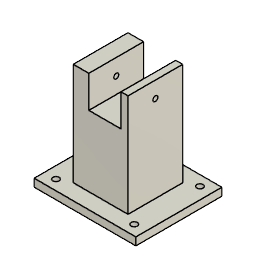
Base_Frotal (Autodesk Fusion 360 design; units mm, degrees)
Autodesk Fusion 360 part; units mm, degrees
sketch "Boceto2" plane through (0, 0, 0) normal (0, 0, 1) x (1, 0, 0)
  line L0 (0, 0) -> (35, 0)
  line L1 (35, 0) -> (35, 35)
  line L2 (35, 35) -> (0, 35)
  line L3 (0, 35) -> (0, 0)
  line L4 (50, -10) -> (-15, -10)
  line L5 (-15, -10) -> (-15, 45)
  line L6 (-15, 45) -> (50, 45)
  line L7 (50, 45) -> (50, -10)
  line L8 (50, -10) -> (-15, 45) construction
  line L9 (-15, -10) -> (50, 45) construction
  line L10 (42.5, 38.5) -> (-7.5, 38.5) construction
  line L11 (-7.5, 38.5) -> (-7.5, -3.5) construction
  line L12 (-7.5, -3.5) -> (42.5, -3.5) construction
  line L13 (42.5, -3.5) -> (42.5, 38.5) construction
  line L14 (42.5, 38.5) -> (-7.5, -3.5) construction
  line L15 (-7.5, 38.5) -> (42.5, -3.5) construction
  circle A0 centre (42.5, 38.5) radius 2
  line L16 (17.5, 45) -> (17.5, -10) construction
  line L17 (-15, 17.5) -> (50, 17.5) construction
  circle A1 centre (-7.5, 38.5) radius 2
  circle A2 centre (-7.5, -3.5) radius 2
  circle A3 centre (42.5, -3.5) radius 2
  point P0 (17.5, 17.5)
  point P1 (17.5, 17.5)
  dimension "d8" = 35
  dimension "d9" = 35
  dimension "d10" = 15
  dimension "d12" = 10
  dimension "d13" = 10
  dimension "d14" = 15
  dimension "d15" = 50
  dimension "d16" = 42
  dimension "d17" = 4
  constraint horizontal L0
  constraint vertical L1
  constraint horizontal L2
  constraint vertical L3
  constraint coincident L0.start L3.end
  constraint horizontal L4
  constraint perpendicular L4 L5
  constraint parallel L4 L6
  constraint parallel L5 L7
  constraint coincident L8 P1
  constraint coincident L9 P1
  constraint horizontal L10
  constraint perpendicular L10 L11
  constraint parallel L10 L12
  constraint parallel L11 L13
  constraint coincident L14 P1
  constraint coincident L15 P1
  constraint coincident P1 P0
  constraint coincident L10.start L13.end
  constraint midpoint L6 L16.start
  constraint midpoint L4 L16.end
  constraint midpoint L5 L17.start
  constraint midpoint L7 L17.end
  constraint symmetric A0 L16 A1
  constraint symmetric A0 L17 A3
  constraint symmetric L17 A1 A2
  measures "d8" distance of L0 L2
  measures "d9" distance of L1 L3
  measures "d10" distance of L3 L5
  measures "d12" distance of L0 L4
  measures "d13" distance of L2 L6
  measures "d14" distance of L1 L7
  measures "d15" distance of L11.end L12.end
  measures "d16" distance of L10.end L11.end
  measures "d17" diameter of A0
extrude "Extruir1" add sketch "Boceto2" along normal blind 70.5 contours L0 L1 L2 L3
sketch "Boceto3" plane through (0, 0, 0) normal (0, -1, 0) x (1, 0, 0)
  line L0 (0, 0) -> (35, 0)
  line L1 (35, 0) -> (35, 70.5)
  line L2 (35, 70.5) -> (0, 70.5)
  line L3 (0, 70.5) -> (0, 0)
  line L4 (0, 70.5) -> (10, 70.5)
  line L5 (10, 70.5) -> (30.5, 70.5)
  line L6 (30.5, 70.5) -> (30.5, 50)
  line L7 (30.5, 50) -> (10, 50)
  line L8 (10, 50) -> (10, 70.5)
  dimension "d3" = 10
  dimension "d4" = 20.5
  dimension "d5" = 20.5
  constraint coincident L2.end L3.start
  constraint perpendicular L1 L4
  constraint horizontal L5
  constraint vertical L6
  constraint horizontal L7
  constraint vertical L8
  measures "d3" distance of L2.end L4.end
  measures "d4" distance of L4.end L5.end
  measures "d5" distance of L4.end L7.end
extrude "Extruir2" cut sketch "Boceto3" against normal blind 35 contours L2 L5 L6 L7 L8
sketch "Boceto4" plane through (0, 0, 50) normal (0, 0, 1) x (-1, 0, 0)
  line L0 (-10, 0) -> (-30.5, 0)
  line L1 (-30.5, 0) -> (-30.5, -35)
  line L2 (-30.5, -35) -> (-10, -35)
  line L3 (-10, -35) -> (-10, 0)
  line L4 (-20.25, -35) -> (-20.25, 0)
  constraint midpoint L2 L4.start
  constraint midpoint L0 L4.end
extrude "Extruir3" add sketch "Boceto2" along normal blind 5
sketch "Boceto5" plane through (35, 0, 0) normal (1, 0, 0) x (0, 1, 0)
  line L0 (0, 5) -> (35, 5)
  line L1 (35, 5) -> (35, 70.5)
  line L2 (35, 70.5) -> (0, 70.5)
  line L3 (0, 70.5) -> (0, 5)
  line L4 (0, 70.5) -> (35, 70.5)
  line L5 (35, 70.5) -> (35, 50)
  line L6 (35, 50) -> (0, 50)
  line L7 (0, 50) -> (0, 70.5)
  circle A0 centre (17.5, 60.25) radius 1.6
  dimension "d20" = 3.2
  constraint horizontal L4
  constraint vertical L5
  constraint horizontal L6
  constraint vertical L7
  constraint coincident L1 L5.end
  constraint coincident L2.end L3.start
  measures "d20" diameter of A0
extrude "Extruir4" cut sketch "Boceto5" against normal blind 45 contours A0
